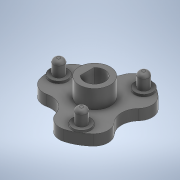
# Autodesk Inventor part: Impeller
Saved by Autodesk Inventor 2020.2 (Build 242310000, 310)
## iProperties
Created: 2020-09-02
Part Number: Impeller
Material: Generic
Document SubType Name: Modeling
Designer: JK
Density: 1 g/cm^3
Appearance: Smooth - Black
Author: JK
Autodesk Inventor part; units mm, degrees
ref_plane "YZ Plane" through (0, 0, 0) normal (1, 0, 0) x (0, 1, 0)
ref_plane "XZ Plane" through (0, 0, 0) normal (0, 1, 0) x (-1, 0, 0)
ref_plane "XY Plane" through (0, 0, 0) normal (0, 0, 1) x (1, 0, 0)
sketch "Sketch1" plane through (0, 0, 0) normal (0, 1, 0) x (-1, 0, 0)
  circle A0 centre (0, 0) radius 2.75
  circle A1 centre (0, 0) radius 12.5
  line L0 (2, 1.8875) -> (2, -1.8875)
  dimension "d0" = 5.5
  dimension "d1" = 2
  dimension "d2" = 25
  constraints: 2 centre point, 2 coincident, 2 end point, 2 point on circle, 1 vertical
  measures "d0" diameter of A0
  measures "d1" distance from line of point (0, 0) L0
  measures "d2" diameter of A1
extrude "Extrusion1" add sketch "Sketch1" along normal blind 3 contours A0 L0 | A1 picked at (2.1064, -0.4926)
sketch "Sketch2" plane through (0, 3, 0) normal (0, 1, 0) x (1, 0, 0)
  circle A0 centre (-10, 0) radius 1.45
  circle A1 centre (0, 0) radius 12.5 projected
  dimension "d5" = 2.9
  dimension "d12" = 10
  constraints: 1 centre point
  measures "d5" diameter of A0
  measures "d12" distance of point (0, 0) A0.centre
extrude "Extrusion2" add sketch "Sketch2" along normal blind 4.5 contours A0
pattern_circular "Circular Pattern1" count 3 over 360 about axis through (0, 0, 0) along (0, 1, 0) of "Extrusion2"
sketch "Sketch3" plane through (0, 3, 0) normal (0, 1, 0) x (1, 0, 0)
  circle A0 centre (0, 0) radius 12.5 projected
  circle A1 centre (12.5, 0) radius 5
  dimension "d13" = 10
  constraints: 1 centre point, 1 horizontal alignment, 1 other
  measures "d13" diameter of A1
extrude "Extrusion3" cut sketch "Sketch3" against normal blind 10 contours A0 A1 | A0 A1 picked at (10.9107, -1.1658) picked at (13.9683, -1.2721)
pattern_circular "Circular Pattern2" count 3 over 360 about axis through (0, 0, 0) along (0, 1, 0) of "Extrusion3"
fillet "Fillet1" radius 4 6 edges at (-1.5074, 1.5, -12.4088) (-9.9926, 1.5, -7.5098) (-1.5074, 1.5, 12.4088) (-9.9926, 1.5, 7.5098) (11.5, 1.5, -4.899) (11.5, 1.5, 4.899)
sketch "Sketch4" plane through (0, 3, 0) normal (0, 1, 0) x (1, 0, 0)
  circle A0 centre (5, -8.6603) radius 1.45 projected
  circle A1 centre (5, -8.6603) radius 2.5
  arc A2 (3.4545, -12.0132) -> (8.6765, -8.9983) centre (0, 0) ccw projected
  constraints: 1 centre point, 1 coincident, 1 tangent
extrude "Extrusion4" add sketch "Sketch4" along normal blind 0.6
pattern_circular "Circular Pattern3" count 3 over 360 about axis through (0, 0, 0) along (0, 1, 0) of "Extrusion4"
sketch "Sketch5" plane through (12.5, 3, 0) normal (0, 1, 0) x (1, 0, 0)
  circle A0 centre (-12.5, 0) radius 2.75
  circle A1 centre (-12.5, 0) radius 4.35
  arc A2 (-14.5, -1.8875) -> (-14.5, 1.8875) centre (-12.5, 0) ccw projected
  arc A3 (-3.6667, 3.3993) -> (-3.8235, 8.9983) centre (-6.6, 6.1188) ccw projected
  arc A4 (-3.8235, 8.9983) -> (-6.25, 10.8253) centre (-12.5, 0) ccw projected
  circle A5 centre (-7.5, 8.6603) radius 2.5 projected
  arc A6 (-6.25, 10.8253) -> (-9.0455, 12.0132) centre (-12.5, 0) ccw projected
  arc A7 (-9.0455, 12.0132) -> (-13.9727, 9.3496) centre (-10.1509, 8.169) ccw projected
  arc A8 (-19.8606, 5.9502) -> (-13.9727, 9.3496) centre (-18.75, 10.8253) ccw projected
  arc A9 (-19.8606, 5.9502) -> (-24.631, 3.0149) centre (-20.7491, 2.0501) ccw projected
  arc A10 (-24.631, 3.0149) -> (-25, 0) centre (-12.5, 0) ccw projected
  circle A11 centre (-22.5, 0) radius 2.5 projected
  arc A12 (-25, 0) -> (-24.631, -3.0149) centre (-12.5, 0) ccw projected
  arc A13 (-24.631, -3.0149) -> (-19.8606, -5.9502) centre (-20.7491, -2.0501) ccw projected
  arc A14 (-13.9727, -9.3496) -> (-19.8606, -5.9502) centre (-18.75, -10.8253) ccw projected
  arc A15 (-13.9727, -9.3496) -> (-9.0455, -12.0132) centre (-10.1509, -8.169) ccw projected
  arc A16 (-9.0455, -12.0132) -> (-6.25, -10.8253) centre (-12.5, 0) ccw projected
  circle A17 centre (-7.5, -8.6603) radius 2.5 projected
  arc A18 (-6.25, -10.8253) -> (-3.8235, -8.9983) centre (-12.5, 0) ccw projected
  arc A19 (-3.8235, -8.9983) -> (-3.6667, -3.3993) centre (-6.6, -6.1188) ccw projected
  arc A20 (-3.6667, 3.3993) -> (-3.6667, -3.3993) centre (0, 0) ccw projected
  arc A21 (-14.5, -1.8875) -> (-14.5, 1.8875) centre (-12.5, 0) ccw projected
  line L0 (-14.5, -1.8875) -> (-14.5, 1.8875) projected
  point P0 (-14.5, -1.8875)
  point P1 (-14.5, 1.8875)
  dimension "d25" = 1.6
  constraints: 2 centre point, 2 coincident, 1 concentric, 1 horizontal alignment, 2 other
  measures "d25" radial gap between concentric circles of A0 A1
extrude "Extrusion5" add sketch "Sketch5" along normal blind 5.14 contours L0 A0 | A1 picked at (-14.6194, -0.4716)
fillet "Fillet2" radius 1 3 edges at (-11.45, 7.5, 0) (5.725, 7.5, -9.916) (5.725, 7.5, 9.916)
sketch "Sketch6" plane through (0, 8.14, 0) normal (0, 1, 0) x (1, 0, 0)
  circle A0 centre (0, 0) radius 4.35 projected
  arc A1 (-2, -1.8875) -> (-2, 1.8875) centre (0, 0) ccw projected
  line L0 (-2, -1.8875) -> (-2, 1.8875) projected
  arc A2 (-2.1, -1.9268) -> (-2.1, 1.9268) centre (0, 0) ccw
  line L1 (-2.1, -1.9268) -> (-2.1, 1.9268)
  dimension "d29" = 0.1
  constraints: 2 end point, 2 point on circle, 1 centre point, 1 other
  measures "d29" radial gap between concentric circles of A2 A1
extrude "Extrusion6" cut sketch "Sketch6" against normal through all contours L1 A2
body "Solid1"
